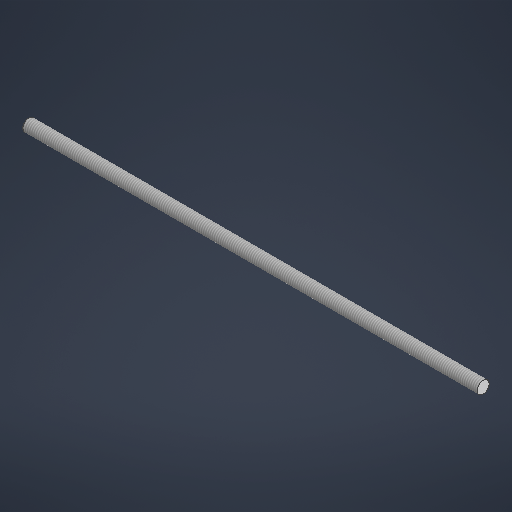
# Autodesk Inventor part: P_Gewindestange_M4_150mm
Saved by Autodesk Inventor 2026 (Build 300175000, 175)
## iProperties
Created: 2025-04-25
Part Number: P_Gewindestange_M4_150mm
Material: Generisch
Document SubType Name: Modeling
Designer: FAL
Density: 1 g/cm^3
Appearance: Vorgabe
Author: FAL
Autodesk Inventor part; units mm, degrees
ref_plane "YZ Plane" through (0, 0, 0) normal (1, 0, 0) x (0, 1, 0)
ref_plane "XZ Plane" through (0, 0, 0) normal (0, 1, 0) x (-1, 0, 0)
ref_plane "XY Plane" through (0, 0, 0) normal (0, 0, 1) x (1, 0, 0)
sketch "Skizze1" plane through (0, 0, 0) normal (0, 0, 1) x (1, 0, 0)
  line L0 (0, 0) -> (150, 0)
  dimension "d0" = 150
  constraints: 2 end point, 1 horizontal
  measures "d0" distance of L0.start L0.end
ref_plane "Arbeitsebene1" through (0, 0, 0) normal (1, 0, 0) x (0, 1, 0)
sketch "Skizze2" plane through (0, 0, 0) normal (1, 0, 0) x (0, 1, 0)
  circle A0 centre (0, 0) radius 2
  dimension "d1" = 4
  constraints: 1 centre point, 1 coincident
  measures "d1" diameter of A0
sweep "Sweeping1" add profiles "Skizze2" path "Skizze1"
thread "Gewinde1"
